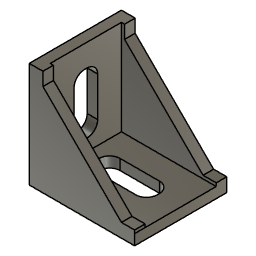
4040A angle bracket v1 (Autodesk Fusion 360 design; units mm, degrees)
Autodesk Fusion 360 part; units mm, degrees
sketch "Sketch1" plane through (0, 0, 0) normal (1, 0, 0) x (0, 1, 0)
  line L0 (17.5, -20) -> (-17.5, -20)
  line L1 (-17.5, -20) -> (-17.5, 20)
  line L2 (-17.5, 20) -> (17.5, 20)
  line L3 (17.5, 20) -> (17.5, -20)
  line L4 (17.5, -20) -> (-17.5, 20) construction
  line L5 (-17.5, -20) -> (17.5, 20) construction
  line L6 (0.5, 11.5) -> (-0.5, 11.5)
  line L7 (-4.5, 7.5) -> (-4.5, -7.5)
  line L8 (-0.5, -11.5) -> (0.5, -11.5)
  line L9 (4.5, -7.5) -> (4.5, 7.5)
  line L10 (4.5, 11.5) -> (-4.5, -11.5) construction
  line L11 (-4.5, 11.5) -> (4.5, -11.5) construction
  arc A0 (-0.5, 11.5) -> (-4.5, 7.5) centre (-0.5, 7.5) ccw
  arc A1 (4.5, 7.5) -> (0.5, 11.5) centre (0.5, 7.5) ccw
  arc A2 (-4.5, -7.5) -> (-0.5, -11.5) centre (-0.5, -7.5) ccw
  arc A3 (0.5, -11.5) -> (4.5, -7.5) centre (0.5, -7.5) ccw
  dimension "d1" = 35
  dimension "d2" = 40
  dimension "d3" = 9
  dimension "d4" = 23
  dimension "d5" = 4
  dimension "d6" = 4
  dimension "d7" = 4
  dimension "d8" = 4
  constraint horizontal L0
  constraint perpendicular L0 L1
  constraint parallel L0 L2
  constraint parallel L1 L3
  constraint coincident L4 origin
  constraint coincident L5 origin
  constraint horizontal L6
  constraint perpendicular L6 L7
  constraint parallel L6 L8
  constraint parallel L7 L9
  constraint coincident L10 origin
  constraint coincident L11 origin
  constraint coincident L11.start L7
  constraint coincident L11.start L6
  constraint tangent L7 A0
  constraint tangent L6 A0
  constraint coincident L10.start L6
  constraint coincident L10.start L9
  constraint tangent L6 A1
  constraint tangent L9 A1
  constraint coincident L10.end L7
  constraint coincident L10.end L8
  constraint tangent L7 A2
  constraint tangent L8 A2
  constraint coincident L11.end L8
  constraint coincident L11.end L9
  constraint tangent L8 A3
  constraint tangent L9 A3
  measures "d1" distance of L1.end L2.end
  measures "d2" distance of L0.end L1.end
  measures "d3" distance of L10.end L11.end
  measures "d4" distance of L11.start L10.end
  measures "d5" radius of A0
  measures "d6" radius of A1
  measures "d7" radius of A2
  measures "d8" radius of A3
extrude "Extrude1" add sketch "Sketch1" along normal blind 4
sketch "Sketch2" plane through (0, 0, -20) normal (0, 0, -1) x (1, 0, 0)
  line L0 (0, 17.5) -> (0, -17.5)
  line L1 (0, -17.5) -> (4, -17.5)
  line L2 (4, -17.5) -> (4, 17.5)
  line L3 (4, 17.5) -> (0, 17.5)
  line L4 (4, -17.5) -> (40, -17.5)
  line L5 (40, -17.5) -> (40, 17.5)
  line L6 (40, 17.5) -> (4, 17.5)
  line L7 (4, -17.5) -> (4, 17.5)
  line L8 (12.5, 4.5) -> (27.5, 4.5)
  line L9 (31.5, 0.5) -> (31.5, -0.5)
  line L10 (27.5, -4.5) -> (12.5, -4.5)
  line L11 (8.5, -0.5) -> (8.5, 0.5)
  line L12 (8.5, 4.5) -> (31.5, -4.5) construction
  line L13 (31.5, 4.5) -> (8.5, -4.5) construction
  arc A0 (27.5, -4.5) -> (31.5, -0.5) centre (27.5, -0.5) ccw
  arc A1 (8.5, -0.5) -> (12.5, -4.5) centre (12.5, -0.5) ccw
  arc A2 (12.5, 4.5) -> (8.5, 0.5) centre (12.5, 0.5) ccw
  arc A3 (31.5, 0.5) -> (27.5, 4.5) centre (27.5, 0.5) ccw
  point P0 (20, -17.5)
  point P1 (20, 0)
  point P2 (20, 0)
  dimension "d11" = 40
  dimension "d13" = 17.5
  dimension "d14" = 20
  dimension "d15" = 23
  dimension "d16" = 9
  dimension "d17" = 4
  dimension "d18" = 4
  dimension "d19" = 4
  dimension "d20" = 4
  constraint horizontal L4
  constraint vertical L5
  constraint horizontal L6
  constraint coincident L1.end L2.start
  constraint coincident L2.end L3.start
  constraint horizontal L8
  constraint perpendicular L8 L9
  constraint parallel L8 L10
  constraint parallel L9 L11
  constraint coincident L12 P2
  constraint coincident L13 P2
  constraint coincident P2 P1
  constraint coincident L12.end L9
  constraint coincident L12.end L10
  constraint tangent L9 A0
  constraint tangent L10 A0
  constraint coincident L13.end L10
  constraint coincident L13.end L11
  constraint tangent L10 A1
  constraint tangent L11 A1
  constraint coincident L12.start L11
  constraint coincident L12.start L8
  constraint tangent L11 A2
  constraint tangent L8 A2
  constraint coincident L13.start L9
  constraint coincident L13.start L8
  constraint tangent L9 A3
  constraint tangent L8 A3
  constraint coincident L4 P0
  measures "d11" distance of L0.end L4.end
  measures "d13" distance of L4 P2
  measures "d14" distance of L5 P2
  measures "d15" distance of L12.end L13.end
  measures "d16" distance of L13.start L12.end
  measures "d17" radius of A0
  measures "d18" radius of A1
  measures "d19" radius of A2
  measures "d20" radius of A3
extrude "Extrude2" add sketch "Sketch2" against normal blind 4 contours L2 L4 L5 L6 L7
sketch "Sketch3" plane through (0, 17.5, 0) normal (0, 1, 0) x (-1, 0, 0)
  line L0 (0, -20) -> (0, 20)
  line L1 (0, 20) -> (-4, 20)
  line L2 (-4, 20) -> (-4, -16)
  line L3 (-4, -16) -> (-40, -16)
  line L4 (-40, -16) -> (-40, -20)
  line L5 (-40, -20) -> (0, -20)
  line L6 (-4, 20) -> (-5.2, 20)
  line L7 (-5.2, -16) -> (-4, -16)
  line L8 (-4, -16) -> (-4, 20)
  line L9 (-40, -16) -> (-5.2, -16)
  line L10 (-5.2, -16) -> (-5.2, -14.8)
  line L11 (-35, -14.8) -> (-40, -14.8)
  line L12 (-40, -14.8) -> (-40, -16)
  line L13 (-35, -14.8) -> (-5.2, 15)
  line L14 (-35, -14.8) -> (6.8148, -14.8) construction
  line L15 (-5.2, 20) -> (-5.2, 15)
  line L16 (-5.2, -14.8) -> (-5.2, -16)
  dimension "d23" = 1.2
  dimension "d24" = 1.2
  dimension "d25" = 45
  dimension "d26" = 5
  constraint horizontal L6
  constraint vertical L15
  constraint horizontal L7
  constraint vertical L8
  constraint coincident L3 L7.start
  constraint coincident L1.end L2.start
  constraint horizontal L9
  constraint vertical L10
  constraint horizontal L11
  constraint vertical L12
  constraint coincident L10.end L15
  constraint coincident L3.end L4.start
  constraint horizontal L14
  constraint collinear L15 L16
  measures "d23" distance of L1.end L6.end
  measures "d24" distance of L3.end L11.end
  measures "d25" angle of L13 L14
  measures "d26" distance of L11.end L11.start
extrude "Extrude3" add sketch "Sketch3" against normal blind 4 contours L2 L3 L6 L7 L8 L9 L11 L12 L13 L15
sketch "Sketch4" plane through (0, -17.5, 0) normal (0, -1, 0) x (1, 0, 0)
  line L0 (0, 20) -> (0, -20)
  line L1 (0, -20) -> (40, -20)
  line L2 (40, -20) -> (40, -16)
  line L3 (40, -16) -> (4, -16)
  line L4 (4, -16) -> (4, 20)
  line L5 (4, 20) -> (0, 20)
  line L6 (4, 20) -> (5.2, 20)
  line L7 (5.2, 20) -> (5.2, 15)
  line L8 (5.2, 15) -> (35, -14.8)
  line L9 (35, -14.8) -> (40, -14.8)
  line L10 (40, -14.8) -> (40, -16)
  dimension "d29" = 1.2
  constraint coincident L4.end L5.start
  constraint perpendicular L4 L6
  constraint perpendicular L6 L7
  constraint perpendicular L0 L9
  constraint coincident L2.end L3.start
  measures "d29" distance of L4.end L6.end
extrude "Extrude4" add sketch "Sketch4" against normal blind 4 contours L3 L4 L6 L7 L8 L9 L10
